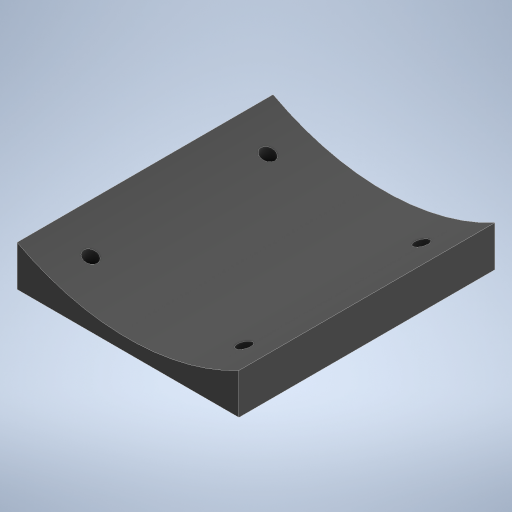
# Autodesk Inventor part: toe_back_buf
Saved by Autodesk Inventor 2024.1 (Build 281209000, 209)
## iProperties
Created: 2024-02-12
Part Number: toe_back_buf
Material: 一般
Document SubType Name: Modeling
Designer: hibik
Density: 1 g/cm^3
Appearance: 既定
Author: hibik
Autodesk Inventor part; units mm, degrees
ref_plane "YZ Plane" through (0, 0, 0) normal (1, 0, 0) x (0, 1, 0)
ref_plane "XZ Plane" through (0, 0, 0) normal (0, 1, 0) x (-1, 0, 0)
ref_plane "XY Plane" through (0, 0, 0) normal (0, 0, 1) x (1, 0, 0)
sketch "スケッチ1" plane through (0, 0, 0) normal (0, 0, 1) x (1, 0, 0)
  line L0 (0, 31) -> (26, 31)
  line L1 (26, 31) -> (26, 0)
  line L2 (26, 0) -> (0, 0)
  line L3 (0, 0) -> (0, 31)
  circle A0 centre (13, 31) radius 27.5
  point P0 (26, 6.7668)
  point P1 (0, 6.7668)
  dimension "d0" = 55
  dimension "d1" = 31
  dimension "d3" = 26
  constraints: 8 end point, 2 parallel, 1 centre point, 1 coincident, 1 horizontal, 1 midpoint, 1 perpendicular
  measures "d0" diameter of A0
  measures "d1" distance from line of L2 A0.centre
  measures "d3" distance between parallel lines of L1 L3
extrude "押し出し1" add sketch "スケッチ1" along normal blind 30 contours A0 L1 L2 L3
sketch "スケッチ2" plane through (0, 0, 0) normal (0, -1, 0) x (1, 0, 0)
  line L0 (26, 0) -> (0, 30)
  line L1 (0, 0) -> (26, 30)
  line L2 (22, 4.6154) -> (4, 4.6154)
  line L3 (4, 4.6154) -> (4, 25.3846)
  line L4 (4, 25.3846) -> (22, 25.3846)
  line L5 (22, 25.3846) -> (22, 4.6154)
  line L6 (26, 0) -> (26, 30) projected
  line L7 (26, 0) -> (0, 0) projected
  line L8 (0, 0) -> (0, 32) projected
  circle A0 centre (22, 4.6154) radius 0.8
  circle A1 centre (4, 4.6154) radius 0.8
  circle A2 centre (4, 25.3846) radius 0.8
  circle A3 centre (22, 25.3846) radius 0.8
  dimension "d6" = 4
  dimension "d7" = 1.6
  dimension "d8" = 1.6
  dimension "d9" = 1.6
  dimension "d10" = 1.6
  constraints: 12 end point, 5 coincident, 5 point on line, 4 centre point, 2 parallel, 1 horizontal, 1 perpendicular
  measures "d6" distance between parallel lines of L6 L5
  measures "d7" diameter of A0
  measures "d8" diameter of A1
  measures "d9" diameter of A2
  measures "d10" diameter of A3
extrude "押し出し2" cut sketch "スケッチ2" against normal through all contours A0 L2 L0 | L0 L5 A0 | L2 A0 L0 | L0 A0 L5 | A3 L5 L1 | L1 L4 A3 | A1 L3 L1 | L1 L2 A1 | L2 L1 A1 | L5 A3 L1 | L1 A3 L4 | L3 A1 L1 | A2 L4 L0 | L0 L3 A2 | A2 L0 L4 | L3 L0 A2
sketch "スケッチ3" plane through (0, 0, 0) normal (0, -1, 0) x (1, 0, 0)
  line L0 (-10, 40) -> (50, 40)
  line L1 (50, 40) -> (50, -10)
  line L2 (50, -10) -> (-10, -10)
  line L3 (-10, -10) -> (-10, 40)
  point P0 (0, 0)
  constraints: 8 end point, 2 parallel, 1 horizontal, 1 perpendicular
extrude "押し出し3" cut sketch "スケッチ3" against normal blind 2
